Fan connector_v1 (Autodesk Fusion 360 design; units mm, degrees)
Autodesk Fusion 360 part; units mm, degrees
sketch "Sketch1" plane through (0, 0, 0) normal (0, 0, 1) x (1, 0, 0) in component "Connector"
  line L0 (6.75, -4.75) -> (-6.75, -4.75)
  line L1 (-6.75, -4.75) -> (-6.75, 4.75)
  line L2 (-6.75, 4.75) -> (6.75, 4.75)
  line L3 (6.75, 4.75) -> (6.75, -4.75)
  line L4 (6.75, -4.75) -> (-6.75, 4.75) construction
  line L5 (-6.75, -4.75) -> (6.75, 4.75) construction
  line L6 (-5.75, 4.75) -> (-2.25, 4.75)
  line L7 (-2.25, 4.75) -> (-2.25, 3.25)
  line L8 (-2.25, 3.25) -> (-5.75, 3.25)
  line L9 (-5.75, 3.25) -> (-5.75, 4.75)
  line L10 (0, 0) -> (0, 4.75) construction
  line L11 (2.25, 3.25) -> (5.75, 3.25)
  line L12 (2.25, 4.75) -> (2.25, 3.25)
  line L13 (5.75, 3.25) -> (5.75, 4.75)
  line L14 (5.75, 4.75) -> (2.25, 4.75)
  line L15 (0, -4.75) -> (0, -0.9) construction
  line L16 (6, -1.9) -> (-6, -1.9)
  line L17 (-6, -1.9) -> (-6, 0.1)
  line L18 (-6, 0.1) -> (6, 0.1)
  line L19 (6, 0.1) -> (6, -1.9)
  line L20 (6, -1.9) -> (-6, 0.1) construction
  line L21 (-6, -1.9) -> (6, 0.1) construction
  line L22 (-5.5, -3.85) -> (-4.5, -3.85)
  line L23 (-4.5, -3.85) -> (-4.5, -2.85)
  line L24 (-4.5, -2.85) -> (-5.5, -2.85)
  line L25 (-5.5, -2.85) -> (-5.5, -3.85)
  line L26 (-3.5, -3.85) -> (-2.5, -3.85)
  line L27 (-2.5, -3.85) -> (-2.5, -2.85)
  line L28 (-2.5, -2.85) -> (-3.5, -2.85)
  line L29 (-3.5, -2.85) -> (-3.5, -3.85)
  line L30 (-1.5, -3.85) -> (-0.5, -3.85)
  line L31 (-0.5, -3.85) -> (-0.5, -2.85)
  line L32 (-0.5, -2.85) -> (-1.5, -2.85)
  line L33 (-1.5, -2.85) -> (-1.5, -3.85)
  line L34 (0.5, -3.85) -> (1.5, -3.85)
  line L35 (1.5, -3.85) -> (1.5, -2.85)
  line L36 (1.5, -2.85) -> (0.5, -2.85)
  line L37 (0.5, -2.85) -> (0.5, -3.85)
  line L38 (2.5, -3.85) -> (3.5, -3.85)
  line L39 (3.5, -3.85) -> (3.5, -2.85)
  line L40 (3.5, -2.85) -> (2.5, -2.85)
  line L41 (2.5, -2.85) -> (2.5, -3.85)
  line L42 (4.5, -3.85) -> (5.5, -3.85)
  line L43 (5.5, -3.85) -> (5.5, -2.85)
  line L44 (5.5, -2.85) -> (4.5, -2.85)
  line L45 (4.5, -2.85) -> (4.5, -3.85)
  line L46 (-5.5, -3.85) -> (-6.75, -3.85) construction
  line L47 (5.5, -3.85) -> (6.75, -3.85) construction
  line L48 (0, -0.9) -> (6, -0.9) construction
  line L49 (-1.5, 1.05) -> (-1.5, 2.05)
  line L50 (4.5, 1.05) -> (4.5, 2.05)
  line L51 (1.5, 2.05) -> (1.5, 1.05)
  line L52 (-0.5, 2.05) -> (-0.5, 1.05)
  line L53 (-3.5, 2.05) -> (-2.5, 2.05)
  line L54 (-2.5, 1.05) -> (-3.5, 1.05)
  line L55 (-2.5, 2.05) -> (-2.5, 1.05)
  line L56 (3.5, 1.05) -> (2.5, 1.05)
  line L57 (1.5, 1.05) -> (0.5, 1.05)
  line L58 (-4.5, 2.05) -> (-4.5, 1.05)
  line L59 (0.5, 1.05) -> (0.5, 2.05)
  line L60 (3.5, 2.05) -> (3.5, 1.05)
  line L61 (-1.5, 2.05) -> (-0.5, 2.05)
  line L62 (-5.5, 2.05) -> (-4.5, 2.05)
  line L63 (5.5, 2.05) -> (5.5, 1.05)
  line L64 (-0.5, 1.05) -> (-1.5, 1.05)
  line L65 (2.5, 1.05) -> (2.5, 2.05)
  line L66 (4.5, 2.05) -> (5.5, 2.05)
  line L67 (-3.5, 1.05) -> (-3.5, 2.05)
  line L68 (5.5, 1.05) -> (4.5, 1.05)
  line L69 (0.5, 2.05) -> (1.5, 2.05)
  line L70 (-4.5, 1.05) -> (-5.5, 1.05)
  line L71 (-5.5, 1.05) -> (-5.5, 2.05)
  line L72 (2.5, 2.05) -> (3.5, 2.05)
  point P0 (0, -0.9)
  dimension "d1" = 13.5
  dimension "d2" = 9.5
  dimension "d3" = 3.5
  dimension "d4" = 1.5
  dimension "d5" = 1
  dimension "d6" = 3.85
  dimension "d7" = 12
  dimension "d8" = 2
  dimension "d9" = 1
  dimension "d10" = 1
  dimension "d11" = 0.9
  dimension "d15" = 2
  dimension "d16" = 0
  constraint horizontal L0
  constraint perpendicular L0 L1
  constraint parallel L0 L2
  constraint parallel L1 L3
  constraint coincident L4 L10.start
  constraint coincident L5 L10.start
  constraint coincident L10.start origin
  constraint horizontal L6
  constraint vertical L7
  constraint horizontal L8
  constraint vertical L9
  constraint coincident L2 L6.start
  constraint midpoint L2 L10.end
  constraint symmetric L6.start L10 L13.end
  constraint symmetric L6.end L10 L12.start
  constraint symmetric L7.end L10 L11.start
  constraint symmetric L8.end L10 L11.end
  constraint midpoint L0 L15.start
  constraint perpendicular L0 L15
  constraint horizontal L16
  constraint perpendicular L16 L17
  constraint parallel L16 L18
  constraint parallel L17 L19
  constraint coincident L20 P0
  constraint coincident L21 P0
  constraint coincident P0 L15.end
  constraint horizontal L22
  constraint vertical L23
  constraint horizontal L24
  constraint vertical L25
  constraint coincident L1 L46.end
  constraint perpendicular L1 L46
  constraint coincident L3 L47.end
  constraint perpendicular L3 L47
  constraint equal L46 L47
  constraint midpoint L19 L48.end
  constraint symmetric L22.start L48 L62.start
  constraint symmetric L22.end L48 L58.start
  constraint symmetric L23.end L48 L58.end
  constraint symmetric L24.end L48 L70.end
  constraint symmetric L26.start L48 L53.start
  constraint symmetric L26.end L48 L53.end
  constraint symmetric L27.end L48 L54.start
  constraint symmetric L28.end L48 L54.end
  constraint symmetric L30.start L48 L49.end
  constraint symmetric L30.end L48 L52.start
  constraint symmetric L31.end L48 L52.end
  constraint symmetric L32.end L48 L49.start
  constraint symmetric L34.start L48 L59.end
  constraint symmetric L34.end L48 L51.start
  constraint symmetric L35.end L48 L51.end
  constraint symmetric L36.end L48 L57.end
  constraint symmetric L38.start L48 L65.end
  constraint symmetric L38.end L48 L60.start
  constraint symmetric L39.end L48 L56.start
  constraint symmetric L40.end L48 L56.end
  constraint symmetric L42.start L48 L50.end
  constraint symmetric L42.end L48 L63.start
  constraint symmetric L43.end L48 L63.end
  constraint symmetric L44.end L48 L50.start
  measures "d1" distance of L1.end L2.end
  measures "d2" distance of L0.end L1.end
  measures "d3" distance of L6.start L6.end
  measures "d4" distance of L6.start L8.end
  measures "d5" distance of L1 L9
  measures "d6" distance of L15.start P0
  measures "d7" distance of L17.end L18.end
  measures "d8" distance of L16.end L17.end
  measures "d9" distance of L22.start L22.end
  measures "d10" distance of L22.start L24.end
  measures "d11" distance of L0 L22
  measures "d21" diameter of L51.start
extrude "Extrude1" add sketch "Sketch1" along normal blind 7 contours L0 L1 L2 L3 L7 L8 L9 L11 L12 L13 makes body 1 in component "Connector"
sketch "Sketch1 (2)" plane through (0, 0, 0) normal (0, 0, 1) x (1, 0, 0) in component "Socket"
  line L0 (4.5, -2.85) -> (4.5, -3.85) construction
  line L1 (4.5, -3.85) -> (5.5, -3.85) construction
  line L2 (5.5, -3.85) -> (5.5, -2.85) construction
  line L3 (5.5, -2.85) -> (4.5, -2.85) construction
  line L4 (0.5, -2.85) -> (0.5, -3.85) construction
  line L5 (0.5, -3.85) -> (1.5, -3.85) construction
  line L6 (1.5, -3.85) -> (1.5, -2.85) construction
  line L7 (1.5, -2.85) -> (0.5, -2.85) construction
  line L8 (-5.5, -2.85) -> (-5.5, -3.85) construction
  line L9 (-5.5, -3.85) -> (-4.5, -3.85) construction
  line L10 (-4.5, -3.85) -> (-4.5, -2.85) construction
  line L11 (-4.5, -2.85) -> (-5.5, -2.85) construction
  line L12 (-5.5, 1.05) -> (-4.5, 1.05) construction
  line L13 (-4.5, 1.05) -> (-4.5, 2.05) construction
  line L14 (-4.5, 2.05) -> (-5.5, 2.05) construction
  line L15 (-5.5, 2.05) -> (-5.5, 1.05) construction
  line L16 (2.5, 2.05) -> (2.5, 1.05) construction
  line L17 (2.5, 1.05) -> (3.5, 1.05) construction
  line L18 (3.5, 1.05) -> (3.5, 2.05) construction
  line L19 (3.5, 2.05) -> (2.5, 2.05) construction
  line L20 (0.5, 2.05) -> (0.5, 1.05) construction
  line L21 (0.5, 1.05) -> (1.5, 1.05) construction
  line L22 (1.5, 1.05) -> (1.5, 2.05) construction
  line L23 (1.5, 2.05) -> (0.5, 2.05) construction
  line L24 (5.5, 1.05) -> (5.5, 2.05) construction
  line L25 (5.5, 2.05) -> (4.5, 2.05) construction
  line L26 (4.5, 2.05) -> (4.5, 1.05) construction
  line L27 (4.5, 1.05) -> (5.5, 1.05) construction
  line L28 (-0.5, 1.05) -> (-0.5, 2.05) construction
  line L29 (-0.5, 2.05) -> (-1.5, 2.05) construction
  line L30 (-1.5, 2.05) -> (-1.5, 1.05) construction
  line L31 (-1.5, 1.05) -> (-0.5, 1.05) construction
  line L32 (-3.5, 1.05) -> (-2.5, 1.05) construction
  line L33 (-2.5, 1.05) -> (-2.5, 2.05) construction
  line L34 (-2.5, 2.05) -> (-3.5, 2.05) construction
  line L35 (-3.5, 2.05) -> (-3.5, 1.05) construction
  line L36 (-1.5, -2.85) -> (-1.5, -3.85) construction
  line L37 (-1.5, -3.85) -> (-0.5, -3.85) construction
  line L38 (-0.5, -3.85) -> (-0.5, -2.85) construction
  line L39 (-0.5, -2.85) -> (-1.5, -2.85) construction
  line L40 (2.5, -2.85) -> (2.5, -3.85) construction
  line L41 (2.5, -3.85) -> (3.5, -3.85) construction
  line L42 (3.5, -3.85) -> (3.5, -2.85) construction
  line L43 (3.5, -2.85) -> (2.5, -2.85) construction
  line L44 (-3.5, -2.85) -> (-3.5, -3.85) construction
  line L45 (-3.5, -3.85) -> (-2.5, -3.85) construction
  line L46 (-2.5, -3.85) -> (-2.5, -2.85) construction
  line L47 (-2.5, -2.85) -> (-3.5, -2.85) construction
  line L48 (6, 0.1) -> (-6, 0.1) construction
  line L49 (-6, 0.1) -> (-6, -1.9) construction
  line L50 (-6, -1.9) -> (6, -1.9) construction
  line L51 (6, -1.9) -> (6, 0.1) construction
  line L52 (-2.25, 3.25) -> (-2.25, 4.75)
  line L53 (-2.25, 4.75) -> (2.25, 4.75)
  line L54 (2.25, 4.75) -> (2.25, 3.25)
  line L55 (2.25, 3.25) -> (5.75, 3.25)
  line L56 (5.75, 3.25) -> (5.75, 4.75)
  line L57 (5.75, 4.75) -> (6.75, 4.75)
  line L58 (6.75, 4.75) -> (6.75, -4.75)
  line L59 (6.75, -4.75) -> (-6.75, -4.75)
  line L60 (-6.75, -4.75) -> (-6.75, 4.75)
  line L61 (-6.75, 4.75) -> (-5.75, 4.75)
  line L62 (-5.75, 4.75) -> (-5.75, 3.25)
  line L63 (-5.75, 3.25) -> (-2.25, 3.25)
  line L64 (-8.25, -6.25) -> (8.25, -6.25)
  line L65 (8.25, -6.25) -> (8.25, 6.25)
  line L66 (8.25, 6.25) -> (-8.25, 6.25)
  line L67 (-8.25, 6.25) -> (-8.25, -6.25)
  line L68 (-8.25, -6.25) -> (8.25, 6.25) construction
  line L69 (8.25, -6.25) -> (-8.25, 6.25) construction
  line L70 (5.5, 1.05) -> (4.5, 2.05) construction
  line L71 (5.5, -3.85) -> (4.5, -2.85) construction
  line L72 (3.5, -3.85) -> (2.5, -2.85) construction
  line L73 (1.5, -3.85) -> (0.5, -2.85) construction
  line L74 (3.5, 1.05) -> (2.5, 2.05) construction
  line L75 (1.5, 1.05) -> (0.5, 2.05) construction
  line L76 (-0.5, 1.05) -> (-1.5, 2.05) construction
  line L77 (-2.5, 1.05) -> (-3.5, 2.05) construction
  line L78 (-4.5, 1.05) -> (-5.5, 2.05) construction
  line L79 (-4.5, -3.85) -> (-5.5, -2.85) construction
  line L80 (-2.5, -3.85) -> (-3.5, -2.85) construction
  line L81 (-0.5, -3.85) -> (-1.5, -2.85) construction
  circle A0 centre (5, 1.55) radius 0.3
  circle A1 centre (3, 1.55) radius 0.3
  circle A2 centre (1, 1.55) radius 0.3
  circle A3 centre (-1, 1.55) radius 0.3
  circle A4 centre (-3, 1.55) radius 0.3
  circle A5 centre (-5, 1.55) radius 0.3
  circle A6 centre (-5, -3.35) radius 0.3
  circle A7 centre (-3, -3.35) radius 0.3
  circle A8 centre (-1, -3.35) radius 0.3
  circle A9 centre (1, -3.35) radius 0.3
  circle A10 centre (3, -3.35) radius 0.3
  circle A11 centre (5, -3.35) radius 0.3
  dimension "d19" = 1.5
  dimension "d20" = 1.5
  dimension "d21" = 0.6
  constraint horizontal L64
  constraint perpendicular L64 L65
  constraint parallel L64 L66
  constraint parallel L65 L67
  constraint coincident L68 origin
  constraint coincident L69 origin
  constraint coincident L24.start L27.end
  constraint coincident L25.end L26.start
  constraint coincident L1.end L2.start
  constraint coincident L0.start L3.end
  constraint coincident L41.end L42.start
  constraint coincident L40.start L43.end
  constraint coincident L5.end L6.start
  constraint coincident L4.start L7.end
  constraint coincident L17.end L18.start
  constraint coincident L16.start L19.end
  constraint coincident L21.end L22.start
  constraint coincident L20.start L23.end
  constraint coincident L28.start L31.end
  constraint coincident L29.end L30.start
  constraint coincident L32.end L33.start
  constraint coincident L34.end L35.start
  constraint coincident L12.end L13.start
  constraint coincident L14.end L15.start
  constraint coincident L9.end L10.start
  constraint coincident L8.start L11.end
  constraint coincident L45.end L46.start
  constraint coincident L44.start L47.end
  constraint coincident L37.end L38.start
  constraint coincident L36.start L39.end
  constraint midpoint L70 A0.centre
  constraint midpoint L74 A1.centre
  constraint midpoint L75 A2.centre
  constraint midpoint L76 A3.centre
  constraint midpoint L77 A4.centre
  constraint midpoint L78 A5.centre
  constraint midpoint L79 A6.centre
  constraint midpoint L80 A7.centre
  constraint midpoint L81 A8.centre
  constraint midpoint L73 A9.centre
  constraint midpoint L72 A10.centre
  constraint midpoint L71 A11.centre
  constraint equal A0 A1
  constraint equal A0 A2
  constraint equal A0 A3
  constraint equal A0 A4
  constraint equal A0 A5
  constraint equal A0 A6
  constraint equal A0 A7
  constraint equal A0 A8
  constraint equal A0 A9
  constraint equal A0 A10
  constraint equal A0 A11
  measures "d19" distance of L59 L64
  measures "d20" distance of L60 L67
  measures "d21" diameter of A0
extrude "Extrude1'" add sketch "Sketch1 (2)" along normal blind 6 separate body contours L64 L65 L66 L67 makes body 2 in component "Socket"
extrude "Extrude2" add sketch "Sketch1 (2)" against normal blind 1 contours L52 L53 L54 L55 L56 L57 L58 L59 L60 L61 L62 L63 | L64 L65 L66 L67 bodies 2 in component "Socket"
move_face "OffsetFaces1" offset -0.15 11 faces at (-0.75, 4.75, 2) (-2.25, 4.25, 4) (-4.5833, 3.25, 2) (-6.4167, 4.75, 2) (-6.75, -1.5833, 2) (3.4167, 3.25, 2) (5.75, 4.25, 4) (2.25, 4.25, 2) (-5.75, 4.25, 2) (6.75, 1.5833, 2) (2.25, -4.75, 2) on bodies 2 in component "Socket"
component "Connector" placed x (1, 0, 0) y (0, 1, 0) z (0, 0, 1) at (0, 0, 0)
component "Socket" placed x (1, 0, 0) y (0, 1, 0) z (0, 0, 1) at (0, 0, 0)
equation "d6 = 2.85 mm + d8 / 2"
equation "d20 = d19"
